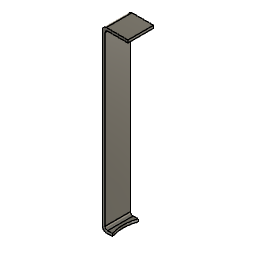
Motor Tube regular v3 (Autodesk Fusion 360 archive; units mm, degrees)
design "Motor Hook"
Autodesk Fusion 360 part; units mm, degrees
sketch "Sketch1" plane through (0, 0, 0) normal (0, 1, 0) x (1, 0, 0)
  line L0 (6, -26.7) -> (-2, -26.7)
  line L1 (-1.2679, -27.7) -> (6, -27.7)
  line L2 (6, -27.7) -> (6, -26.7)
  line L3 (-3, -25.7) -> (-3, 40)
  line L4 (-4, 39.268) -> (-4, -26.2)
  line L5 (-2.5, 42) -> (0, 42)
  line L6 (0, 42) -> (0, 41)
  line L7 (0, 41) -> (-2, 41)
  arc A0 (-2, 41) -> (-3, 40) centre (-2, 40) ccw
  arc A1 (-3, -25.7) -> (-2, -26.7) centre (-2, -25.7) ccw
  line L8 (-1.2679, -27.7) -> (-2.5, -27.7)
  line L9 (-4, 39.268) -> (-4, 40.5)
  arc A2 (-2.5, 42) -> (-4, 40.5) centre (-2.5, 40.5) ccw
  arc A3 (-4, -26.2) -> (-2.5, -27.7) centre (-2.5, -26.2) ccw
  dimension "d6" = 67.7
  dimension "d7" = 1
  dimension "d8" = 1
  dimension "d9" = 1
  dimension "d12" = 10
  dimension "d13" = 1.5
  dimension "d14" = 1.5
  constraint horizontal L0
  constraint horizontal L1
  constraint vertical L2
  constraint vertical L3
  constraint vertical L4
  constraint horizontal L5
  constraint vertical L6
  constraint horizontal L7
  constraint tangent L3 A0
  constraint tangent L7 A0
  constraint tangent L0 A1
  constraint tangent L3 A1
  constraint perpendicular L4 L8
  constraint perpendicular L5 L9
  constraint tangent L5 A2
  constraint tangent L9 A2
  constraint tangent L8 A3
  constraint tangent L4 A3
  measures "d6" distance of L0 L7
  measures "d7" distance of L0 L1
  measures "d8" distance of L3 L4
  measures "d9" distance of L5 L7
  measures "d12" distance of L2 L4
  measures "d13" radius of A2
  measures "d14" radius of A3
extrude "Extrude1" add sketch "Sketch1" along normal blind 10
sketch "Sketch2" plane through (0, 0, -41) normal (0, 0, 1) x (-1, 0, 0)
  line L0 (2, 0) -> (0, 0)
  line L1 (0, 0) -> (0, -10)
  line L2 (0, -10) -> (2, -10)
  line L3 (2, -10) -> (2, 0)
  line L4 (0, 0) -> (0, -10)
  line L5 (-13.3846, -5) -> (0, -10) construction
  line L6 (-13.3846, -5) -> (0, 0) construction
  arc A0 (0, -10) -> (0, 0) centre (-13.3846, -5) ccw
  arc A1 (0, -10) -> (0, 0) centre (-13.3846, -5) ccw
  dimension "d19" = 14.288
  dimension "d20" = 14.288
  constraint coincident L1.end L2.start
  constraint coincident L0.end L1.start
  constraint coincident L5.start L6.start
  measures "d19" distance of L5.start L1.end
  measures "d20" distance of L0.end L5.start
extrude "Extrude2" cut sketch "Sketch2" against normal blind 10 contours L1 L4 A0 A1
equation "d6 = 80 mm - 12.3 mm"

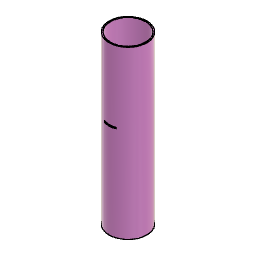
design "Motor mount tube"
Autodesk Fusion 360 part; units mm, degrees
sketch "Sketch1" plane through (0, 0, 0) normal (0, 0, 1) x (1, 0, 0)
  circle A0 centre (0, 0) radius 15
  circle A1 centre (0, 0) radius 16
  dimension "d1" = 30
  dimension "d2" = 32
  constraint coincident A0.centre A1.centre
  measures "d1" diameter of A0
  measures "d2" diameter of A1
extrude "Extrude1" add sketch "Sketch1" along normal blind 140
sketch "Sketch2" plane through (0, 0, 0) normal (0, 1, 0) x (1, 0, 0)
  line L0 (0, 0) -> (0, -78.88) construction
  line L1 (5, -79.88) -> (-5, -79.88)
  line L2 (-5, -79.88) -> (-5, -78.88)
  line L3 (5, -78.88) -> (5, -79.88)
  line L4 (5, -79.88) -> (0, -78.88) construction
  line L5 (-5, -79.88) -> (0, -78.88) construction
  line L6 (-5, -79.88) -> (5, -79.88)
  line L7 (5, -79.88) -> (5, -78.88)
  line L8 (5, -78.88) -> (-5, -78.88)
  line L9 (-5, -78.88) -> (-5, -79.88)
  point P0 (0, -78.88)
  dimension "d5" = 78.88
  constraint coincident L0.start origin
  constraint vertical L0
  constraint horizontal L1
  constraint perpendicular L1 L2
  constraint parallel L2 L3
  constraint coincident L4 P0
  constraint coincident L5 P0
  constraint coincident P0 L0.end
  constraint horizontal L6
  constraint vertical L7
  constraint horizontal L8
  constraint vertical L9
  measures "d5" distance of L0.start P0
extrude "Extrude2" cut sketch "Sketch2" along normal through all and the other way through all
sketch "Sketch3" plane through (0, 0, 0) normal (0, 0, -1) x (1, 0, 0)
  circle A0 centre (0, 0) radius 15
  circle A1 centre (0, 0) radius 16
  circle A2 centre (0, 0) radius 16
  circle A3 centre (0, 0) radius 15
  constraint coincident A0.centre A1.centre
extrude "Extrude3" add sketch "Sketch3" along normal blind 1.25
equation "d5 = 80 mm - 1.12 mm"

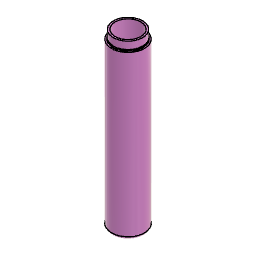
design "Cesaroni 29Pro 2G casing"
Autodesk Fusion 360 part; units mm, degrees
sketch "Sketch1" plane through (0, 0, 0) normal (0, 0, 1) x (1, 0, 0)
  circle A0 centre (0, 0) radius 14.2875
  dimension "d1" = 28.575
  constraint coincident A0.centre origin
  measures "d1" diameter of A0
extrude "Extrude1" add sketch "Sketch1" along normal blind 142.24 thin wall 3.175 on the right open curves A0
extrude "Extrude2" add sketch "Sketch1" along normal blind 3.175
fillet "Fillet1" radius 2.5 1 edges at (-13.3206, -5.1666, 0)
sketch "Sketch2" plane through (0, 0, 142.24) normal (0, 0, 1) x (-1, 0, 0)
  circle A0 centre (0, 0) radius 11.1125
  circle A1 centre (0, 0) radius 14.2875
  circle A2 centre (0, 0) radius 12.7
  dimension "d15" = 25.4
  constraint coincident A0.centre A1.centre
  measures "d15" diameter of A2
extrude "Extrude3" add sketch "Sketch2" along normal mid plane 12.7 contours A2
sketch "Sketch3" plane through (0, 0, 142.24) normal (0, 0, 1) x (-1, 0, 0)
  circle A0 centre (0, 0) radius 14.2875
  circle A1 centre (0, 0) radius 12.7
  circle A2 centre (0, 0) radius 13
  dimension "d17" = 0.3
extrude "Extrude4" cut sketch "Sketch3" against normal blind 1 contours A0
sketch "Sketch4" plane through (0, 0, 0) normal (0, 0, -1) x (1, 0, 0)
  circle A0 centre (0, 0) radius 11.7875
  circle A1 centre (0, 0) radius 10
  dimension "d18" = 20
  constraint coincident A0.centre A1.centre
  measures "d18" diameter of A1
extrude "Extrude5" cut sketch "Sketch4" against normal blind 10 contours A1

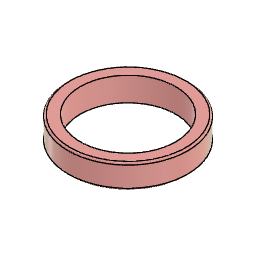
design "Cesaroni 29Pro 2G regular closure"
Autodesk Fusion 360 part; units mm, degrees
sketch "Sketch1" plane through (0, 0, 0) normal (0, 0, 1) x (1, 0, 0)
  circle A0 centre (0, 0) radius 15.875
  circle A1 centre (0, 0) radius 12.7
  dimension "d1" = 31.75
  dimension "d2" = 25.4
  constraint coincident A0.centre A1.centre
  constraint concentric A0 A1
  measures "d1" diameter of A0
  measures "d2" diameter of A1
extrude "Extrude1" add sketch "Sketch1" along normal blind 6.35
fillet "Fillet1" radius 0.5 2 edges at (-14.8007, -5.7406, 0) (-14.8007, -5.7406, 6.35)
